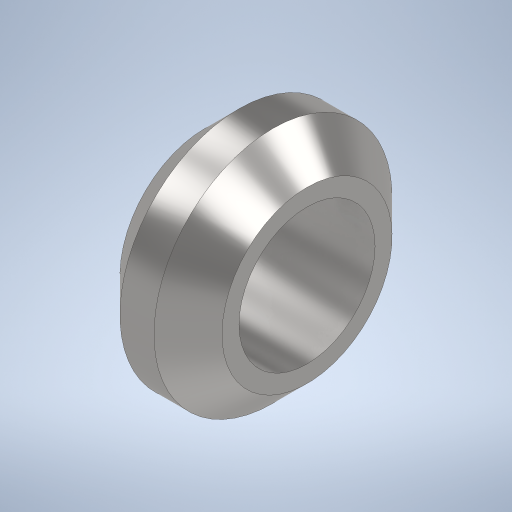
# Autodesk Inventor part: pieza 1-27
Saved by Autodesk Inventor 2024 (Build 280153000, 153)
## iProperties
Created: 2024-10-05
Part Number: pieza 1-27
Material: Iron, Malleable
Document SubType Name: Modeling
Designer: katam
Density: 7.15 g/cm^3
Appearance: Semi-Polished
Author: katam
Autodesk Inventor part; units mm, degrees
ref_plane "YZ Plane" through (0, 0, 0) normal (1, 0, 0) x (0, 1, 0)
ref_plane "XZ Plane" through (0, 0, 0) normal (0, 1, 0) x (-1, 0, 0)
ref_plane "XY Plane" through (0, 0, 0) normal (0, 0, 1) x (1, 0, 0)
sketch "Sketch1" plane through (0, 0, 0) normal (0, 0, 1) x (1, 0, 0)
  line L0 (0, 0) -> (11.8926, 0)
  line L1 (3.9297, 0) -> (3.9297, 5)
  line L2 (3.9297, 5) -> (5.9297, 7)
  line L3 (5.9297, 7) -> (7.9297, 7)
  line L4 (7.9297, 7) -> (9.9297, 5)
  line L5 (9.9297, 5) -> (9.9297, 0)
  line L6 (0.8799, 7) -> (12.9795, 7) construction
  line L7 (6.9297, 9.4343) -> (6.9297, -2.3254) construction
  line L8 (5.9297, 7) -> (5.9463, 0)
  line L9 (7.9297, 7) -> (7.9297, 0)
  point P0 (6.9297, 7)
  point P1 (3.9297, 2.5)
  point P2 (9.9297, 2.5)
  point P3 (6.9297, 7)
  dimension "d0" = 2
  dimension "d1" = 45
  dimension "d3" = 45
  dimension "d4" = 14
  dimension "d6" = 3
  dimension "d7" = 3
  constraints: 20 end point, 7 point on line, 5 midpoint, 2 horizontal, 2 perpendicular, 2 vertical
  measures "d0" distance of L2.end L3.end
  measures "d1" angle of L6 L2
  measures "d3" angle of L6 L4
  measures "d4" diameter of point (6.93, 7) L0
  measures "d6" distance between parallel lines of L5 L7
  measures "d7" distance between parallel lines of L1 L7
revolve "Revolution1" add sketch "Sketch1" angle 360 about axis through (0, 0, 0) along (1, 0, 0)
sketch "Sketch2" plane through (9.9297, 0, 0) normal (1, 0, 0) x (0, 0, -1)
  circle A0 centre (0, 0) radius 4
  dimension "d9" = 8
  constraints: 1 centre point, 1 coincident
  measures "d9" diameter of A0
extrude "Extrusion1" cut sketch "Sketch2" against normal blind 10
body "Solid1"
